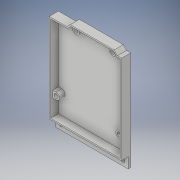
# Autodesk Inventor part: Arduino+Support
Saved by Autodesk Inventor 2019 (Build 230136000, 136)
## iProperties
Created: 2019-02-13
Part Number: Arduino+Support
Material: Générique
Document SubType Name: Modeling
Designer: Quentin
Density: 1 g/cm^3
Appearance: Par défaut
Author: Quentin
Autodesk Inventor part; units mm, degrees
ref_plane "YZ Plane" through (0, 0, 0) normal (1, 0, 0) x (0, 1, 0)
ref_plane "XZ Plane" through (0, 0, 0) normal (0, 1, 0) x (-1, 0, 0)
ref_plane "XY Plane" through (0, 0, 0) normal (0, 0, 1) x (1, 0, 0)
sketch "Esquisse8" plane through (0, 0, 0) normal (0, 0, 1) x (1, 0, 0)
  line L0 (0, 66.04) -> (0, 0)
  line L1 (0, 0) -> (0, 66.04)
  line L2 (12.954, 66.04) -> (0, 66.04)
  line L3 (0, 66.04) -> (12.954, 66.04)
  line L4 (48.26, 68.58) -> (15.494, 68.58)
  line L5 (12.954, 66.04) -> (15.494, 68.58)
  line L6 (50.8, 66.04) -> (48.26, 68.58)
  line L7 (15.494, 68.58) -> (48.26, 68.58)
  line L8 (48.26, 68.58) -> (50.8, 66.04)
  line L9 (53.34, 0) -> (53.34, 66.04)
  line L10 (50.8, 66.04) -> (53.34, 66.04)
  line L11 (53.34, 66.04) -> (53.34, 0)
  line L12 (53.34, 0) -> (0, 0)
  circle A0 centre (2.54, 15.24) radius 1.5875
  circle A1 centre (2.54, 15.24) radius 1.5875
  circle A2 centre (50.8, 13.97) radius 1.5875
  circle A3 centre (50.8, 13.97) radius 1.5875
  circle A4 centre (45.72, 66.04) radius 1.5875
  circle A5 centre (45.72, 66.04) radius 1.5875
  circle A6 centre (17.78, 66.04) radius 1.5875
  circle A7 centre (17.78, 66.04) radius 1.5875
  line L13 (15.0798, 69.58) -> (48.6742, 69.58)
  line L14 (51.2142, 67.04) -> (48.6742, 69.58)
  line L15 (51.2142, 67.04) -> (54.34, 67.04)
  line L16 (54.34, -1) -> (54.34, 67.04)
  line L17 (54.34, -1) -> (-1, -1)
  line L18 (-1, -1) -> (-1, 67.04)
  line L19 (-1, 67.04) -> (12.5398, 67.04)
  line L20 (12.5398, 67.04) -> (15.0798, 69.58)
  dimension "d59" = 1
  dimension "d60" = 1
  dimension "d61" = 1
  dimension "d62" = 1
  dimension "d63" = 1
  dimension "d64" = 1
  dimension "d65" = 1
  constraints: 42 end point, 8 centre point, 7 parallel, 4 coincident, 3 collinear, 2 perpendicular, 1 vertical
  measures "d59" distance between parallel lines of L7 L13
  measures "d60" distance between parallel lines of L6 L14
  measures "d61" distance between parallel lines of L10 L15
  measures "d62" distance between parallel lines of L9 L16
  measures "d63" distance between parallel lines of L12 L17
  measures "d64" distance between parallel lines of L0 L18
  measures "d65" distance between parallel lines of L5 L20
extrude "Extrusion5" add sketch "Esquisse8" along normal blind 7 contours L2 L5 L4 L6 L10 L9 L12 L0 | L13 L14 L15 L16 L17 L18 L19 L20
shell "Coque1" thickness 1 removed faces 1 at (23.8943, 31.957, 7)
sketch "Esquisse10" plane through (0, 0, 1) normal (0, 0, 1) x (1, 0, 0)
  arc A0 (0, 14.7465) -> (0, 15.7335) centre (2.54, 15.24) ccw projected
  line L0 (2.54, 17.8275) -> (0, 17.8275)
  arc A1 (53.34, 14.4635) -> (53.34, 13.4765) centre (50.8, 13.97) ccw projected
  line L1 (50.8, 16.5575) -> (53.34, 16.5575)
  line L2 (50.8, 11.3825) -> (53.34, 11.3825)
  arc A2 (45.2265, 68.58) -> (46.2135, 68.58) centre (45.72, 66.04) ccw projected
  line L3 (43.1325, 66.04) -> (43.1325, 68.58)
  line L4 (48.3075, 66.04) -> (48.3075, 68.58)
  circle A3 centre (2.54, 15.24) radius 2.5875
  line L5 (0, 17.8275) -> (0, 12.6525)
  line L6 (0, 15.7335) -> (0, 66.04) projected
  line L7 (53.34, 16.5575) -> (53.34, 11.3825)
  line L8 (53.34, 66.04) -> (53.34, 14.4635) projected
  line L9 (43.1325, 68.58) -> (48.3075, 68.58)
  line L10 (18.2735, 68.58) -> (45.2265, 68.58) projected
  circle A4 centre (45.72, 66.04) radius 1.5875 projected
  circle A5 centre (45.72, 66.04) radius 2.5875
  circle A6 centre (50.8, 13.97) radius 1.5875 projected
  circle A7 centre (50.8, 13.97) radius 2.5875
  line L11 (2.54, 12.6525) -> (0, 12.6525)
  line L12 (0, 0) -> (0, 14.7465) projected
  constraints: 18 end point, 5 point on circle, 5 tangent, 3 coincident, 3 collinear, 3 horizontal, 2 centre point, 2 concentric, 2 vertical, 1 perpendicular, 1 vertical alignment, 3 other
extrude "Extrusion6" add sketch "Esquisse10" along normal blind 4.35 contours L5 L0 A0 | L7 A1 | A1 L1 L7 | L7 L2 A1 | L9 A2 | A2 L3 L9 | L9 L4 A2
sketch "Esquisse11" plane through (0, 0, 7) normal (0, 0, 1) x (1, 0, 0)
  arc A0 (0, 14.7465) -> (2.54, 17.8275) centre (2.54, 15.24) ccw projected
  line L0 (2.54, 12.6525) -> (0, 12.6525)
  line L1 (0, 0) -> (0, 14.7465) projected
  line L2 (0, 12.6525) -> (0, 14.7465)
  circle A1 centre (2.54, 15.24) radius 2.5875
  constraints: 4 end point, 1 centre point, 1 coincident, 1 collinear, 1 concentric, 1 horizontal, 1 point on circle, 1 tangent
extrude "Extrusion7" add sketch "Esquisse11" against normal blind 6 contours A0 L0 L1
sketch "Esquisse12" plane through (0, 0, 0) normal (0, 0, -1) x (-1, 0, 0)
  line L0 (-54.34, -1) -> (1, -1) projected
  line L1 (1, -1) -> (1, -9)
  line L2 (1, -9) -> (-54.34, -9)
  line L3 (-54.34, -9) -> (-54.34, -1)
  point P0 (0, 0)
  dimension "d80" = 8
  constraints: 6 end point, 1 parallel, 1 perpendicular, 1 vertical
  measures "d80" distance of L0.end L1.end
extrude "Extrusion8" add sketch "Esquisse12" against normal blind 2
sketch "Esquisse13" plane through (0, 0, 2) normal (0, 0, 1) x (1, 0, 0)
  line L0 (-1, -9) -> (54.34, -9) projected
  line L1 (-1, -9) -> (3, -9)
  line L2 (3, -9) -> (3, -1.5792)
  line L3 (-1, -9) -> (-1, 67.04) projected
  line L4 (-1, -9) -> (-1, -5)
  line L5 (-1, -5) -> (3, -5)
  line L6 (26.67, -9) -> (26.67, -6.1659)
  point P0 (0, 0)
  point P1 (50.34, -5)
  dimension "d83" = 4
  dimension "d84" = 4
  constraints: 10 end point, 3 point on line, 2 perpendicular, 1 coincident, 1 midpoint, 1 symmetric about line, 1 vertical
  measures "d83" distance of L0.start L1.end
  measures "d84" distance of L0.start L4.end
hole "Perçage2" at (3, -5, 2) at (50.34, -5, 2) direction (0, 0, -1) diameter 3 end through all
sketch "Esquisse14" plane through (0, 0, 7) normal (0, 0, 1) x (1, 0, 0)
  line L0 (0, 0) -> (0, 12.6525) projected
  line L1 (0, 15.7335) -> (0, 17.8275) projected
  line L2 (0, 12.6525) -> (0, 15.7335)
  arc A0 (2.54, 12.6525) -> (0, 15.7335) centre (2.54, 15.24) ccw projected
  line L3 (0, 12.6525) -> (2.54, 12.6525)
  arc A1 (2.54, 12.6525) -> (0, 15.7335) centre (2.54, 15.24) ccw
  circle A2 centre (2.54, 15.24) radius 1.5875
  circle A3 centre (50.8, 13.97) radius 1.5875 projected
  circle A4 centre (50.8, 13.97) radius 1.5875
  arc A5 (53.34, 14.4635) -> (53.34, 13.4765) centre (50.8, 13.97) ccw
  line L4 (53.34, 66.04) -> (53.34, 14.4635) projected
  line L5 (53.34, 14.4635) -> (53.34, 13.4765)
  arc A6 (48.3075, 66.04) -> (46.2135, 68.58) centre (45.72, 66.04) ccw projected
  line L6 (45.2073, 68.58) -> (46.2135, 68.58)
  circle A7 centre (45.72, 66.04) radius 1.5875
  circle A8 centre (45.72, 66.04) radius 1.5875 projected
  arc A9 (45.2265, 68.58) -> (46.2135, 68.58) centre (45.72, 66.04) ccw
  circle A10 centre (17.78, 66.04) radius 1.5875 projected
  circle A11 centre (17.78, 66.04) radius 1.5875
  arc A12 (17.2865, 68.58) -> (18.2735, 68.58) centre (17.78, 66.04) ccw
  arc A13 (17.2865, 68.58) -> (18.2735, 68.58) centre (17.78, 66.04) ccw projected
  line L7 (17.2865, 68.58) -> (18.2735, 68.58)
  constraints: 10 end point, 8 centre point, 8 coincident, 8 point on circle, 3 horizontal, 2 collinear, 2 point on line, 1 concentric, 1 tangent
extrude "Extrusion9" cut sketch "Esquisse14" against normal blind 1.65 contours L2 A0 L3 | L5 A5
sketch "Esquisse15" plane through (0, 0, 7) normal (0, 0, 1) x (1, 0, 0)
  circle A0 centre (17.78, 66.04) radius 1.5875 projected
  circle A1 centre (17.78, 66.04) radius 1.5875
  arc A2 (17.2865, 68.58) -> (18.2735, 68.58) centre (17.78, 66.04) ccw
  line L0 (15.494, 68.58) -> (17.2865, 68.58) projected
  line L1 (17.2865, 68.58) -> (18.2735, 68.58)
  circle A3 centre (45.72, 66.04) radius 1.5875 projected
  circle A4 centre (45.72, 66.04) radius 1.5875
  arc A5 (45.2265, 68.58) -> (46.2135, 68.58) centre (45.72, 66.04) ccw
  line L2 (18.2735, 68.58) -> (45.2265, 68.58) projected
  arc A6 (45.2265, 68.58) -> (46.2135, 68.58) centre (45.72, 66.04) ccw projected
  line L3 (45.2265, 68.58) -> (46.2135, 68.58)
  point P0 (0, 0)
  constraints: 5 end point, 4 centre point, 4 coincident, 4 point on circle, 1 collinear, 1 horizontal
extrude "Extrusion10" cut sketch "Esquisse15" against normal blind 1.65
